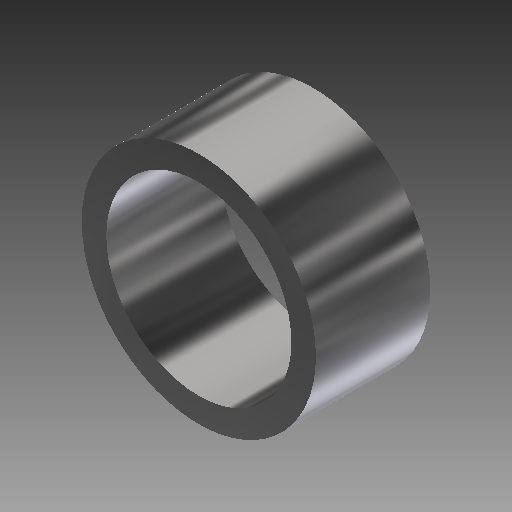
# Autodesk Inventor part: Separator_do_widelca
Saved by Autodesk Inventor 2017 (Build 210142000, 142)
## iProperties
Created: 2016-01-12
Part Number: Separator_do_widelca
Material: Stal, węglowa
Document SubType Name: Modeling
Designer: graaapsik
Density: 7.87 g/cm^3
Appearance: Częściowo polerowany
Mass: 5.75701 g
Surface Area: 9.86963 cm^2
Volume: 0.731514 cm^3
Author: graaapsik
Autodesk Inventor part; units mm, degrees
ref_plane "YZ Plane" through (0, 0, 0) normal (1, 0, 0) x (0, 1, 0)
ref_plane "XZ Plane" through (0, 0, 0) normal (0, 1, 0) x (-1, 0, 0)
ref_plane "XY Plane" through (0, 0, 0) normal (0, 0, 1) x (1, 0, 0)
sketch "Szkic1" plane through (0, 0, 0) normal (0, 0, 1) x (1, 0, 0)
  circle A0 centre (0, 0) radius 8.6
  dimension "d0" = 17.2
  constraints: 1 centre point, 1 coincident
  measures "d0" diameter of A0
extrude "Wyciągnięcie proste1" add sketch "Szkic1" along normal mid plane 8.4
sketch "Szkic2" plane through (0, 0, 4.2) normal (0, 0, 1) x (1, 0, 0)
  circle A0 centre (0, 0) radius 8.6 projected
  constraints: 1 coincident
hole "Otwór1" at (0, 0, 4.2) direction (0, 0, -1) diameter 13.6 end through all
